test2 (Autodesk Fusion 360 design; units mm, degrees)
Autodesk Fusion 360 part; units mm, degrees
sketch "Sketch1" plane through (0, 0, 0) normal (0, 1, 0) x (1, 0, 0) in component "Component"
  circle A0 centre (0, 0) radius 250
  dimension "d7" = 500
  constraint coincident A0.centre origin
  measures "d7" diameter of A0
extrude "Extrude1" add sketch "Sketch1" along normal blind 1500 in component "Component"
sketch "Sketch2" plane through (0, 0, 0) normal (0, 0, 1) x (1, 0, 0) in component "Component"
  circle A0 centre (0, 175) radius 20
  line L0 (0, 0) -> (0, 1500) construction
  circle A1 centre (0, 875) radius 20
  dimension "d10" = 40
  dimension "d11" = 1500
  dimension "d13" = 175
  dimension "d14" = 40
  dimension "d15" = 700
  constraint coincident L0.start origin
  constraint vertical L0
  measures "d10" diameter of A0
  measures "d11" distance of L0.start L0.end
  measures "d13" distance of L0.start A0.centre
  measures "d14" diameter of A1
  measures "d15" distance of A0.centre A1.centre
extrude "Extrude2" cut sketch "Sketch2" along normal blind 475 in component "Component"
sketch "Sketch3" plane through (0, 0, 0) normal (0, -1, 0) x (1, 0, 0) in component "Component"
  circle A0 centre (0, 0) radius 250
  circle A1 centre (0, 0) radius 20
  dimension "d18" = 40
  constraint coincident A0.centre A1.centre
  measures "d18" diameter of A1
extrude "Extrude3" cut sketch "Sketch3" against normal blind 1700 contours A1 in component "Component"
component "Component" placed x (1, 0, 0) y (0, 1, 0) z (0, 0, 1) at (0, 0, 0)
